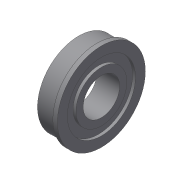
# Autodesk Inventor part: RoundBearing-1-2-inch
Saved by Autodesk Inventor 2013 SP1 (Build 170176100, 176)
## iProperties
Created: 2013-11-18
Part Number: RoundBearing-1-2-inch
Material: Generic
Document SubType Name: Modeling
Designer: robotics
Density: 1 g/cm^3
Author: robotics
Autodesk Inventor part; units mm, degrees
ref_plane "YZ Plane" through (0, 0, 0) normal (1, 0, 0) x (0, 1, 0)
ref_plane "XZ Plane" through (0, 0, 0) normal (0, 1, 0) x (-1, 0, 0)
ref_plane "XY Plane" through (0, 0, 0) normal (0, 0, 1) x (1, 0, 0)
sketch "Sketch1" plane through (0, 0, 0) normal (0, 0, 1) x (1, 0, 0)
  line L0 (0, 14.2875) -> (6.35, 14.2875)
  line L1 (6.35, 14.2875) -> (6.35, 15.2875)
  line L2 (6.35, 15.2875) -> (7.9248, 15.2875)
  line L3 (7.9248, 15.2875) -> (7.9248, 6.35)
  line L4 (7.9248, 6.35) -> (0, 6.35)
  line L5 (0, 6.35) -> (0, 14.2875)
  line L6 (0, 0) -> (7.9248, 0)
  line L7 (0, 11.85) -> (1, 11.85)
  line L8 (1, 11.85) -> (1, 8.85)
  line L9 (1, 8.85) -> (0, 8.85)
  line L10 (0, 8.85) -> (0, 11.85)
  line L11 (7.9248, 8.85) -> (6.9248, 8.85)
  line L12 (6.9248, 8.85) -> (6.9248, 11.85)
  line L13 (6.9248, 11.85) -> (7.9248, 11.85)
  line L14 (7.9248, 11.85) -> (7.9248, 8.85)
  dimension "d0" = 7.9248
  dimension "d2" = 12.7
  dimension "d3" = 28.575
  dimension "d4" = 1.5748
  dimension "d5" = 1
  dimension "d7" = 1
  dimension "d8" = 3
  dimension "d9" = 2.5
  constraints: 30 end point, 8 parallel, 4 perpendicular, 3 horizontal, 3 point on line, 2 horizontal alignment, 1 collinear, 1 vertical alignment
  measures "d0" distance of L3.end L4.end
  measures "d2" diameter of L4 L6
  measures "d3" diameter of L0 L6
  measures "d4" distance between parallel lines of L3 L1
  measures "d5" distance of L0.end L1.end
  measures "d7" distance of L11.start L11.end
  measures "d8" distance of L11.end L12.end
  measures "d9" distance between parallel lines of L4 L11
revolve "Revolution1" add sketch "Sketch1" angle 360 about axis through (0, 0, 0) along (1, 0, 0) contours L0 L1 L2 L3 L13 L12 L11 L4 L5 L9 L8 L7
body "Solid1"
